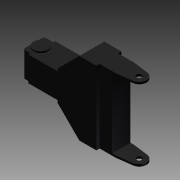
# Autodesk Inventor part: ForeArm
Saved by Autodesk Inventor 2012 (Build 160160000, 160)
## iProperties
Created: 2013-02-21
Part Number: ForeArm
Material: Default
Document SubType Name: Modeling
Designer: Andrew
Density: 1 g/cm^3
Author: Andrew
Autodesk Inventor part; units mm, degrees
ref_plane "YZ Plane" through (0, 0, 0) normal (1, 0, 0) x (0, 1, 0)
ref_plane "XZ Plane" through (0, 0, 0) normal (0, 1, 0) x (-1, 0, 0)
ref_plane "XY Plane" through (0, 0, 0) normal (0, 0, 1) x (1, 0, 0)
sketch "Sketch1" plane through (0, 0, 0) normal (0, 0, 1) x (1, 0, 0)
  circle A0 centre (-141.2963, -27.3767) radius 11
  line L0 (-141.2963, -11.3767) -> (-149.2963, -11.3767)
  line L1 (-152.2963, -14.3767) -> (-152.2963, -27.3767)
  line L2 (-152.2963, -27.3767) -> (-152.2963, -40.3767)
  line L3 (-141.2963, -11.3767) -> (-138.2963, -11.3767)
  line L4 (-138.2963, -11.3767) -> (-138.2963, -8.3767)
  line L5 (-138.2963, -8.3767) -> (-70.2823, -8.3767)
  line L6 (-141.2963, -46.3767) -> (-70.2823, -46.3767)
  line L7 (-141.2963, -46.3767) -> (-141.2963, -43.3767)
  line L8 (-141.2963, -43.3767) -> (-149.2963, -43.3767)
  arc A1 (-149.2963, -11.3767) -> (-152.2963, -14.3767) centre (-149.2963, -14.3767) ccw
  arc A2 (-152.2963, -40.3767) -> (-149.2963, -43.3767) centre (-149.2963, -40.3767) ccw
  line L9 (-23.7963, -41.3767) -> (-13.2963, -41.3767)
  line L10 (-13.2963, -41.3767) -> (10.1436, -38.2818)
  arc A3 (10.1436, -38.2818) -> (10.1436, -16.4717) centre (8.7037, -27.3767) ccw
  line L11 (10.1436, -16.4717) -> (-13.2963, -13.3767)
  line L12 (-13.2963, -13.3767) -> (-37.5536, -13.3767)
  circle A4 centre (8.7037, -27.3767) radius 4
  line L13 (-37.5536, -13.3767) -> (-37.5536, -8.3767)
  line L14 (-37.5536, -8.3767) -> (-70.2823, -8.3767)
  line L15 (-70.2823, -46.3767) -> (-37.5536, -46.3767)
  line L16 (-37.5536, -46.3767) -> (-37.5536, -41.3767)
  line L17 (-23.7963, -41.3767) -> (-37.5536, -41.3767)
  dimension "d18" = 22
  dimension "d20" = 16
  dimension "d22" = 3
  dimension "d27" = 3
  constraints: 36 end point, 6 point on circle, 5 perpendicular, 4 centre point, 4 tangent, 2 equal length, 2 vertical, 1 equal radius, 1 horizontal alignment, 2 other
  measures "d20" distance of point (-141.296, -27.377) L0.start
  measures "d22" distance of L0.start L3.end
  measures "d27" radius of A1
extrude "Extrusion6" add sketch "Sketch1" along normal mid plane 111.5 contours A0 | L1 A1 L0 L3 L4 L5 L14 L13 L12 L11 A3 L10 L9 L17 L16 L15 L6 L7 L8 A2 L2
sketch "Sketch5" plane through (-138.2963, -8.3767, 55.75) normal (0, 1, 0) x (1, 0, 0)
  line L0 (100.7426, 0) -> (100.7426, 111.5) projected
  line L1 (100.7426, 0) -> (100.7426, 3)
  line L2 (100.7426, 3) -> (159.7547, 3)
  line L3 (100.7426, 111.5) -> (100.7426, 108.5)
  line L4 (100.7426, 108.5) -> (159.7547, 108.5)
  line L5 (159.7547, 108.5) -> (159.7547, 3)
  line L6 (100.7426, 3) -> (100.7426, 108.5)
  line L7 (157.9988, 3) -> (119.4988, 3)
  line L8 (119.4988, 3) -> (119.4988, 108.5)
  point P0 (138.2963, 55.75)
  dimension "d32" = 3
  dimension "d33" = 3
  dimension "d34" = 38.5
  constraints: 16 end point, 5 point on line, 3 perpendicular, 2 parallel
  measures "d32" distance of L0.start L1.end
  measures "d33" distance of L0.end L3.end
  measures "d34" distance of L7.start L7.end
extrude "Extrusion7" cut sketch "Sketch5" against normal blind 105.5 contours L8 L4 L5 L2
sketch "Sketch6" plane through (-138.2963, -8.3767, 55.75) normal (0, 1, 0) x (1, 0, 0)
  line L0 (0, 0) -> (100.7426, 0) projected
  line L1 (100.7426, 111.5) -> (0, 111.5) projected
  line L2 (-11, 0) -> (0, 0) projected
  line L3 (0, 0) -> (0, 111.5) projected
  line L4 (0, 111.5) -> (-11, 111.5) projected
  line L5 (-11, 0) -> (-11, 111.5) projected
  line L6 (125, 3) -> (119.4988, 3) projected
  line L7 (119.4988, 3) -> (119.4988, 108.5) projected
  line L8 (119.4988, 108.5) -> (125, 108.5) projected
  line L9 (125, 108.5) -> (125, 111.5) projected
  line L10 (125, 111.5) -> (100.7426, 111.5) projected
  line L11 (100.7426, 0) -> (100.7426, 111.5) projected
  line L12 (100.7426, 0) -> (125, 0) projected
  line L13 (125, 0) -> (125, 3) projected
  line L14 (-14, 0) -> (-11, 0) projected
  line L15 (-11, 0) -> (-11, 111.5) projected
  line L16 (-11, 111.5) -> (-14, 111.5) projected
  line L17 (-14, 0) -> (-14, 111.5) projected
  line L18 (-14, 0) -> (-14, 111.5) projected
  line L19 (-14, 0) -> (-14, 111.5) projected
  line L20 (-14, 55.75) -> (-3, 55.75)
  line L21 (-3, 55.75) -> (-3, 74.75)
  line L22 (-3, 74.75) -> (-14, 74.75)
  line L23 (-3, 55.75) -> (-3, 36.75)
  line L24 (-3, 36.75) -> (-14, 36.75)
  line L25 (-11, 55.75) -> (42, 55.75)
  line L26 (42, 55.75) -> (42, 78.75)
  line L27 (42, 78.75) -> (74.75, 111.5)
  line L28 (-3, 74.75) -> (42, 74.75)
  line L29 (42, 55.75) -> (42, 32.75)
  line L30 (42, 32.75) -> (74.75, 0)
  line L31 (-3, 36.75) -> (42, 36.75)
  line L32 (74.75, 111.5) -> (-14, 111.5)
  line L33 (-14, 111.5) -> (-14, 74.75)
  line L34 (-14, 36.75) -> (-14, 0)
  line L35 (-14, 0) -> (74.75, 0)
  point P0 (138.2963, 55.75)
  dimension "d37" = 11
  dimension "d38" = 19
  dimension "d39" = 19
  dimension "d40" = 53
  dimension "d41" = 23
  dimension "d42" = 135
  dimension "d43" = 23
  constraints: 32 end point, 11 perpendicular, 7 point on line, 3 collinear, 2 midpoint, 1 parallel
  measures "d37" distance of L20.start L20.end
  measures "d38" distance of L20.end L21.end
  measures "d39" distance of L20.end L23.end
  measures "d40" distance of L25.start L25.end
  measures "d41" distance of L25.end L26.end
  measures "d42" angle of L26 L27
  measures "d43" distance of L25.end L29.end
extrude "Extrusion8" cut sketch "Sketch6" against normal blind 105.5 contours L3 L31 L29 L30 L0 | L2 L5 L24 L31 L3 | L14 L17 L24 L5 | L28 L22 L5 L4 L3 | L3 L1 L27 L26 L28 | L22 L17 L16 L5
extrude "Extrusion9" add sketch "Sketch1" along normal mid plane 42 contours A0
body "Solid2"
